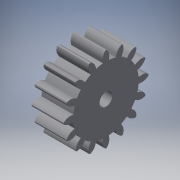
# Autodesk Inventor part: smallergear
Saved by Autodesk Inventor 2018 (Build 220112000, 112)
## iProperties
Created: 2017-10-26
Part Number: smallergear
Material: Generic
Document SubType Name: Modeling
Designer: kcmat
Density: 1 g/cm^3
Appearance: Default
Author: kcmat
Autodesk Inventor part; units mm, degrees
ref_plane "YZ Plane" through (0, 0, 0) normal (1, 0, 0) x (0, 1, 0)
ref_plane "XZ Plane" through (0, 0, 0) normal (0, 1, 0) x (-1, 0, 0)
ref_plane "XY Plane" through (0, 0, 0) normal (0, 0, 1) x (1, 0, 0)
sketch "Sketch1" plane through (0, 0, 0) normal (1, 0, 0) x (0, 1, 0)
  line L0 (1.2701, 13.8679) -> (1.1652, 12.6686)
  line L1 (-1.2699, 13.8679) -> (-1.1639, 12.6567)
  line L2 (-1.1639, 12.6567) -> (-1.1635, 12.6526)
  line L3 (1.1652, 12.6686) -> (1.1638, 12.6522)
  line L4 (-1.1635, 12.6521) -> (-1.1635, 12.6526)
  line L5 (1.1638, 12.6522) -> (1.1638, 12.6521)
  line L6 (1.2701, 13.8679) -> (1.2701, 15.0719) construction
  arc A0 (-0.2778, 16.4478) -> (-1.2699, 13.8679) centre (1.9291, 14.1185) ccw
  arc A1 (1.2701, 13.8679) -> (0.2675, 16.4502) centre (-2.5564, 13.8679) ccw
  arc A2 (0.2675, 16.4502) -> (-0.2778, 16.4478) centre (0.0001, 15.2082) ccw
  circle A3 centre (0, 0) radius 12.7
  line L7 (1.1638, 12.6521) -> (1.1638, 12.6466)
  line L8 (-1.1635, 12.6521) -> (-1.163, 12.6466)
  arc A4 (1.1638, 12.6466) -> (-1.163, 12.6466) centre (0, 0) ccw
  line L9 (-4.1336, 13.2984) -> (-3.7716, 12.1502)
  line L10 (-6.4802, 12.3263) -> (-5.9188, 11.2479)
  line L11 (-5.9188, 11.2479) -> (-5.9169, 11.2442)
  line L12 (-3.7716, 12.1502) -> (-3.7666, 12.1344)
  line L13 (-3.7666, 12.1344) -> (-3.7666, 12.1343)
  line L14 (-5.9167, 11.2437) -> (-5.9169, 11.2442)
  line L15 (-5.9167, 11.2437) -> (-5.9142, 11.2389)
  line L16 (-3.7666, 12.1343) -> (-3.7645, 12.1293)
  arc A5 (-3.7645, 12.1293) -> (-5.9142, 11.2389) centre (0, 0) ccw
  line L17 (-4.1336, 13.2984) -> (-4.5943, 14.4106) construction
  arc A6 (-6.551, 15.0895) -> (-6.4802, 12.3263) centre (-3.6206, 13.782) ccw
  arc A7 (-4.1336, 13.2984) -> (-6.048, 15.3003) centre (-7.6688, 11.834) ccw
  arc A8 (-6.048, 15.3003) -> (-6.551, 15.0895) centre (-5.8198, 14.0505) ccw
  line L18 (-8.908, 10.7042) -> (-8.1341, 9.782)
  line L19 (-10.7041, 8.9082) -> (-9.7726, 8.1266)
  line L20 (-9.7726, 8.1266) -> (-9.7695, 8.124)
  line L21 (-8.1341, 9.782) -> (-8.1235, 9.7693)
  line L22 (-8.1235, 9.7693) -> (-8.1235, 9.7693)
  line L23 (-9.7691, 8.1236) -> (-9.7695, 8.124)
  line L24 (-9.7691, 8.1236) -> (-9.7649, 8.1201)
  line L25 (-8.1235, 9.7693) -> (-8.1196, 9.7654)
  arc A9 (-8.1196, 9.7654) -> (-9.7649, 8.1201) centre (0, 0) ccw
  line L26 (-8.908, 10.7042) -> (-9.7593, 11.5555) construction
  arc A10 (-11.8268, 11.4339) -> (-10.7041, 8.9082) centre (-8.6192, 11.3474) ccw
  arc A11 (-8.908, 10.7042) -> (-11.4429, 11.8212) centre (-11.6138, 7.9985) ccw
  arc A12 (-11.4429, 11.8212) -> (-11.8268, 11.4339) centre (-10.7537, 10.7539) ccw
  line L27 (-12.3263, 6.4805) -> (-11.2584, 5.9246)
  line L28 (-13.2983, 4.1338) -> (-12.1387, 3.7682)
  line L29 (-12.1387, 3.7682) -> (-12.1348, 3.767)
  line L30 (-11.2584, 5.9246) -> (-11.2437, 5.917)
  line L31 (-11.2437, 5.917) -> (-11.2436, 5.9169)
  line L32 (-12.1343, 3.7668) -> (-12.1348, 3.767)
  line L33 (-12.1343, 3.7668) -> (-12.129, 3.7652)
  line L34 (-11.2436, 5.9169) -> (-11.2386, 5.9148)
  arc A13 (-11.2386, 5.9148) -> (-12.129, 3.7652) centre (0, 0) ccw
  line L35 (-12.3263, 6.4805) -> (-13.4385, 6.9412) construction
  arc A14 (-15.3021, 6.0376) -> (-13.2983, 4.1338) centre (-12.3056, 7.1852) ccw
  arc A15 (-12.3263, 6.4805) -> (-15.0956, 6.5424) centre (-13.7906, 2.9452) ccw
  arc A16 (-15.0956, 6.5424) -> (-15.3021, 6.0376) centre (-14.0505, 5.82) ccw
  line L36 (-13.8679, 1.2701) -> (-12.6686, 1.1652)
  line L37 (-13.8679, -1.2699) -> (-12.6567, -1.1639)
  line L38 (-12.6567, -1.1639) -> (-12.6526, -1.1635)
  line L39 (-12.6686, 1.1652) -> (-12.6522, 1.1638)
  line L40 (-12.6522, 1.1638) -> (-12.6521, 1.1638)
  line L41 (-12.6521, -1.1635) -> (-12.6526, -1.1635)
  line L42 (-12.6521, -1.1635) -> (-12.6466, -1.163)
  line L43 (-12.6521, 1.1638) -> (-12.6466, 1.1638)
  arc A17 (-12.6466, 1.1638) -> (-12.6466, -1.163) centre (0, 0) ccw
  line L44 (-13.8679, 1.2701) -> (-15.0719, 1.2701) construction
  arc A18 (-16.4478, -0.2778) -> (-13.8679, -1.2699) centre (-14.1185, 1.9291) ccw
  arc A19 (-13.8679, 1.2701) -> (-16.4502, 0.2675) centre (-13.8679, -2.5564) ccw
  arc A20 (-16.4502, 0.2675) -> (-16.4478, -0.2778) centre (-15.2082, 0.0001) ccw
  line L45 (-13.2984, -4.1336) -> (-12.1502, -3.7716)
  line L46 (-12.3263, -6.4802) -> (-11.2479, -5.9188)
  line L47 (-11.2479, -5.9188) -> (-11.2442, -5.9169)
  line L48 (-12.1502, -3.7716) -> (-12.1344, -3.7666)
  line L49 (-12.1344, -3.7666) -> (-12.1343, -3.7666)
  line L50 (-11.2437, -5.9167) -> (-11.2442, -5.9169)
  line L51 (-11.2437, -5.9167) -> (-11.2389, -5.9142)
  line L52 (-12.1343, -3.7666) -> (-12.1293, -3.7645)
  arc A21 (-12.1293, -3.7645) -> (-11.2389, -5.9142) centre (0, 0) ccw
  line L53 (-13.2984, -4.1336) -> (-14.4106, -4.5943) construction
  arc A22 (-15.0895, -6.551) -> (-12.3263, -6.4802) centre (-13.782, -3.6206) ccw
  arc A23 (-13.2984, -4.1336) -> (-15.3003, -6.048) centre (-11.834, -7.6688) ccw
  arc A24 (-15.3003, -6.048) -> (-15.0895, -6.551) centre (-14.0505, -5.8198) ccw
  line L54 (-10.7042, -8.908) -> (-9.782, -8.1341)
  line L55 (-8.9082, -10.7041) -> (-8.1266, -9.7726)
  line L56 (-8.1266, -9.7726) -> (-8.124, -9.7695)
  line L57 (-9.782, -8.1341) -> (-9.7693, -8.1235)
  line L58 (-9.7693, -8.1235) -> (-9.7693, -8.1235)
  line L59 (-8.1236, -9.7691) -> (-8.124, -9.7695)
  line L60 (-8.1236, -9.7691) -> (-8.1201, -9.7649)
  line L61 (-9.7693, -8.1235) -> (-9.7654, -8.1196)
  arc A25 (-9.7654, -8.1196) -> (-8.1201, -9.7649) centre (0, 0) ccw
  line L62 (-10.7042, -8.908) -> (-11.5555, -9.7593) construction
  arc A26 (-11.4339, -11.8268) -> (-8.9082, -10.7041) centre (-11.3474, -8.6192) ccw
  arc A27 (-10.7042, -8.908) -> (-11.8212, -11.4429) centre (-7.9985, -11.6138) ccw
  arc A28 (-11.8212, -11.4429) -> (-11.4339, -11.8268) centre (-10.7539, -10.7537) ccw
  line L63 (-6.4805, -12.3263) -> (-5.9246, -11.2584)
  line L64 (-4.1338, -13.2983) -> (-3.7682, -12.1387)
  line L65 (-3.7682, -12.1387) -> (-3.767, -12.1348)
  line L66 (-5.9246, -11.2584) -> (-5.917, -11.2437)
  line L67 (-5.917, -11.2437) -> (-5.9169, -11.2436)
  line L68 (-3.7668, -12.1343) -> (-3.767, -12.1348)
  line L69 (-3.7668, -12.1343) -> (-3.7652, -12.129)
  line L70 (-5.9169, -11.2436) -> (-5.9148, -11.2386)
  arc A29 (-5.9148, -11.2386) -> (-3.7652, -12.129) centre (0, 0) ccw
  line L71 (-6.4805, -12.3263) -> (-6.9412, -13.4385) construction
  arc A30 (-6.0376, -15.3021) -> (-4.1338, -13.2983) centre (-7.1852, -12.3056) ccw
  arc A31 (-6.4805, -12.3263) -> (-6.5424, -15.0956) centre (-2.9452, -13.7906) ccw
  arc A32 (-6.5424, -15.0956) -> (-6.0376, -15.3021) centre (-5.82, -14.0505) ccw
  line L72 (-1.2701, -13.8679) -> (-1.1652, -12.6686)
  line L73 (1.2699, -13.8679) -> (1.1639, -12.6567)
  line L74 (1.1639, -12.6567) -> (1.1635, -12.6526)
  line L75 (-1.1652, -12.6686) -> (-1.1638, -12.6522)
  line L76 (-1.1638, -12.6522) -> (-1.1638, -12.6521)
  line L77 (1.1635, -12.6521) -> (1.1635, -12.6526)
  line L78 (1.1635, -12.6521) -> (1.163, -12.6466)
  line L79 (-1.1638, -12.6521) -> (-1.1638, -12.6466)
  arc A33 (-1.1638, -12.6466) -> (1.163, -12.6466) centre (0, 0) ccw
  line L80 (-1.2701, -13.8679) -> (-1.2701, -15.0719) construction
  arc A34 (0.2778, -16.4478) -> (1.2699, -13.8679) centre (-1.9291, -14.1185) ccw
  arc A35 (-1.2701, -13.8679) -> (-0.2675, -16.4502) centre (2.5564, -13.8679) ccw
  arc A36 (-0.2675, -16.4502) -> (0.2778, -16.4478) centre (-0.0001, -15.2082) ccw
  line L81 (4.1336, -13.2984) -> (3.7716, -12.1502)
  line L82 (6.4802, -12.3263) -> (5.9188, -11.2479)
  line L83 (5.9188, -11.2479) -> (5.9169, -11.2442)
  line L84 (3.7716, -12.1502) -> (3.7666, -12.1344)
  line L85 (3.7666, -12.1344) -> (3.7666, -12.1343)
  line L86 (5.9167, -11.2437) -> (5.9169, -11.2442)
  line L87 (5.9167, -11.2437) -> (5.9142, -11.2389)
  line L88 (3.7666, -12.1343) -> (3.7645, -12.1293)
  arc A37 (3.7645, -12.1293) -> (5.9142, -11.2389) centre (0, 0) ccw
  line L89 (4.1336, -13.2984) -> (4.5943, -14.4106) construction
  arc A38 (6.551, -15.0895) -> (6.4802, -12.3263) centre (3.6206, -13.782) ccw
  arc A39 (4.1336, -13.2984) -> (6.048, -15.3003) centre (7.6688, -11.834) ccw
  arc A40 (6.048, -15.3003) -> (6.551, -15.0895) centre (5.8198, -14.0505) ccw
  line L90 (8.908, -10.7042) -> (8.1341, -9.782)
  line L91 (10.7041, -8.9082) -> (9.7726, -8.1266)
  line L92 (9.7726, -8.1266) -> (9.7695, -8.124)
  line L93 (8.1341, -9.782) -> (8.1235, -9.7693)
  line L94 (8.1235, -9.7693) -> (8.1235, -9.7693)
  line L95 (9.7691, -8.1236) -> (9.7695, -8.124)
  line L96 (9.7691, -8.1236) -> (9.7649, -8.1201)
  line L97 (8.1235, -9.7693) -> (8.1196, -9.7654)
  arc A41 (8.1196, -9.7654) -> (9.7649, -8.1201) centre (0, 0) ccw
  line L98 (8.908, -10.7042) -> (9.7593, -11.5555) construction
  arc A42 (11.8268, -11.4339) -> (10.7041, -8.9082) centre (8.6192, -11.3474) ccw
  arc A43 (8.908, -10.7042) -> (11.4429, -11.8212) centre (11.6138, -7.9985) ccw
  arc A44 (11.4429, -11.8212) -> (11.8268, -11.4339) centre (10.7537, -10.7539) ccw
  line L99 (12.3263, -6.4805) -> (11.2584, -5.9246)
  line L100 (13.2983, -4.1338) -> (12.1387, -3.7682)
  line L101 (12.1387, -3.7682) -> (12.1348, -3.767)
  line L102 (11.2584, -5.9246) -> (11.2437, -5.917)
  line L103 (11.2437, -5.917) -> (11.2436, -5.9169)
  line L104 (12.1343, -3.7668) -> (12.1348, -3.767)
  line L105 (12.1343, -3.7668) -> (12.129, -3.7652)
  line L106 (11.2436, -5.9169) -> (11.2386, -5.9148)
  arc A45 (11.2386, -5.9148) -> (12.129, -3.7652) centre (0, 0) ccw
  line L107 (12.3263, -6.4805) -> (13.4385, -6.9412) construction
  arc A46 (15.3021, -6.0376) -> (13.2983, -4.1338) centre (12.3056, -7.1852) ccw
  arc A47 (12.3263, -6.4805) -> (15.0956, -6.5424) centre (13.7906, -2.9452) ccw
  arc A48 (15.0956, -6.5424) -> (15.3021, -6.0376) centre (14.0505, -5.82) ccw
  line L108 (13.8679, -1.2701) -> (12.6686, -1.1652)
  line L109 (13.8679, 1.2699) -> (12.6567, 1.1639)
  line L110 (12.6567, 1.1639) -> (12.6526, 1.1635)
  line L111 (12.6686, -1.1652) -> (12.6522, -1.1638)
  line L112 (12.6522, -1.1638) -> (12.6521, -1.1638)
  line L113 (12.6521, 1.1635) -> (12.6526, 1.1635)
  line L114 (12.6521, 1.1635) -> (12.6466, 1.163)
  line L115 (12.6521, -1.1638) -> (12.6466, -1.1638)
  arc A49 (12.6466, -1.1638) -> (12.6466, 1.163) centre (0, 0) ccw
  line L116 (13.8679, -1.2701) -> (15.0719, -1.2701) construction
  arc A50 (16.4478, 0.2778) -> (13.8679, 1.2699) centre (14.1185, -1.9291) ccw
  arc A51 (13.8679, -1.2701) -> (16.4502, -0.2675) centre (13.8679, 2.5564) ccw
  arc A52 (16.4502, -0.2675) -> (16.4478, 0.2778) centre (15.2082, -0.0001) ccw
  line L117 (13.2984, 4.1336) -> (12.1502, 3.7716)
  line L118 (12.3263, 6.4802) -> (11.2479, 5.9188)
  line L119 (11.2479, 5.9188) -> (11.2442, 5.9169)
  line L120 (12.1502, 3.7716) -> (12.1344, 3.7666)
  line L121 (12.1344, 3.7666) -> (12.1343, 3.7666)
  line L122 (11.2437, 5.9167) -> (11.2442, 5.9169)
  line L123 (11.2437, 5.9167) -> (11.2389, 5.9142)
  line L124 (12.1343, 3.7666) -> (12.1293, 3.7645)
  arc A53 (12.1293, 3.7645) -> (11.2389, 5.9142) centre (0, 0) ccw
  line L125 (13.2984, 4.1336) -> (14.4106, 4.5943) construction
  arc A54 (15.0895, 6.551) -> (12.3263, 6.4802) centre (13.782, 3.6206) ccw
  arc A55 (13.2984, 4.1336) -> (15.3003, 6.048) centre (11.834, 7.6688) ccw
  arc A56 (15.3003, 6.048) -> (15.0895, 6.551) centre (14.0505, 5.8198) ccw
  line L126 (10.7042, 8.908) -> (9.782, 8.1341)
  line L127 (8.9082, 10.7041) -> (8.1266, 9.7726)
  line L128 (8.1266, 9.7726) -> (8.124, 9.7695)
  line L129 (9.782, 8.1341) -> (9.7693, 8.1235)
  line L130 (9.7693, 8.1235) -> (9.7693, 8.1235)
  line L131 (8.1236, 9.7691) -> (8.124, 9.7695)
  line L132 (8.1236, 9.7691) -> (8.1201, 9.7649)
  line L133 (9.7693, 8.1235) -> (9.7654, 8.1196)
  arc A57 (9.7654, 8.1196) -> (8.1201, 9.7649) centre (0, 0) ccw
  line L134 (10.7042, 8.908) -> (11.5555, 9.7593) construction
  arc A58 (11.4339, 11.8268) -> (8.9082, 10.7041) centre (11.3474, 8.6192) ccw
  arc A59 (10.7042, 8.908) -> (11.8212, 11.4429) centre (7.9985, 11.6138) ccw
  arc A60 (11.8212, 11.4429) -> (11.4339, 11.8268) centre (10.7539, 10.7537) ccw
  line L135 (6.4805, 12.3263) -> (5.9246, 11.2584)
  line L136 (4.1338, 13.2983) -> (3.7682, 12.1387)
  line L137 (3.7682, 12.1387) -> (3.767, 12.1348)
  line L138 (5.9246, 11.2584) -> (5.917, 11.2437)
  line L139 (5.917, 11.2437) -> (5.9169, 11.2436)
  line L140 (3.7668, 12.1343) -> (3.767, 12.1348)
  line L141 (3.7668, 12.1343) -> (3.7652, 12.129)
  line L142 (5.9169, 11.2436) -> (5.9148, 11.2386)
  arc A61 (5.9148, 11.2386) -> (3.7652, 12.129) centre (0, 0) ccw
  line L143 (6.4805, 12.3263) -> (6.9412, 13.4385) construction
  arc A62 (6.0376, 15.3021) -> (4.1338, 13.2983) centre (7.1852, 12.3056) ccw
  arc A63 (6.4805, 12.3263) -> (6.5424, 15.0956) centre (2.9452, 13.7906) ccw
  arc A64 (6.5424, 15.0956) -> (6.0376, 15.3021) centre (5.82, 14.0505) ccw
  circle A65 centre (0, 0) radius 2.5
  point P0 (41.2581, -1.1642)
  dimension "d1" = 25.4
  dimension "d4" = 360
  dimension "d6" = 5
  constraints: 288 end point, 130 point on circle, 66 centre point, 16 point on line, 2 coincident, 1 vertical, 481 other
  measures "d1" diameter of A3
  measures "d6" diameter of A65
extrude "Extrusion1" add sketch "Sketch1" along normal blind 12.4
body "Solid1"
